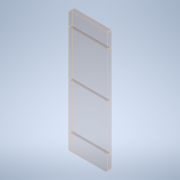
# Autodesk Inventor part: 関節3_上板
Saved by Autodesk Inventor 2021 (Build 250183000, 183)
## iProperties
Created: 2022-02-02
Part Number: 関節3_上板
Material: ポリカーボネート、スモーク
Document SubType Name: Modeling
Designer: hirohumi
Density: 1.2 g/cm^3
Appearance: ポリカーボネート - スモーク
Author: hirohumi
Autodesk Inventor part; units mm, degrees
ref_plane "YZ Plane" through (0, 0, 0) normal (1, 0, 0) x (0, 1, 0)
ref_plane "XZ Plane" through (0, 0, 0) normal (0, 1, 0) x (-1, 0, 0)
ref_plane "XY Plane" through (0, 0, 0) normal (0, 0, 1) x (1, 0, 0)
sketch "スケッチ1" plane through (0, 0, 0) normal (0, 0, 1) x (1, 0, 0)
  line L0 (25.5, 80) -> (-25.5, 80)
  line L1 (-25.5, 80) -> (-25.5, 60.7746)
  line L2 (-25.5, -80) -> (25.5, -80)
  line L3 (25.5, -80) -> (25.5, -60.7746)
  line L4 (25.5, 80) -> (-25.5, -80) construction
  line L5 (-25.5, 80) -> (25.5, -80) construction
  arc A0 (-25.5, 0.7746) -> (-25.5, -0.7746) centre (-26.9, 0) ccw construction
  arc A1 (-25.5, 60.7746) -> (-25.5, 59.2254) centre (-26.9, 60) ccw construction
  arc A2 (-25.5, -59.2254) -> (-25.5, -60.7746) centre (-26.9, -60) ccw construction
  arc A3 (25.5, 0.7746) -> (25.5, -0.7746) centre (26.9, 0) ccw
  arc A4 (25.5, 60.7746) -> (25.5, 59.2254) centre (26.9, 60) ccw
  arc A5 (25.5, -60.7746) -> (25.5, -59.2254) centre (26.9, -60) ccw construction
  arc A6 (-25.5, 59.2254) -> (-25.5, 60.7746) centre (-26.9, 60) ccw
  line L6 (-25.5, 60.7746) -> (-25.5, 59.2254) construction
  line L7 (-25.5, 59.2254) -> (-25.5, 0.7746)
  arc A7 (-25.5, -0.7746) -> (-25.5, 0.7746) centre (-26.9, 0) ccw
  line L8 (-25.5, -0.7746) -> (-25.5, -59.2254)
  line L9 (-25.5, 0.7746) -> (-25.5, -0.7746) construction
  line L10 (-25.5, -59.2254) -> (-25.5, -60.7746) construction
  line L11 (-25.5, -60.7746) -> (-25.5, -80)
  arc A8 (-25.5, -60.7746) -> (-25.5, -59.2254) centre (-26.9, -60) ccw
  arc A9 (25.5, -59.2254) -> (25.5, -60.7746) centre (26.9, -60) ccw
  line L12 (25.5, -60.7746) -> (25.5, -59.2254) construction
  line L13 (25.5, -59.2254) -> (25.5, -0.7746)
  arc A10 (25.5, -0.7746) -> (25.5, 0.7746) centre (26.9, 0) ccw construction
  line L14 (25.5, -0.7746) -> (25.5, 0.7746) construction
  line L15 (25.5, 0.7746) -> (25.5, 59.2254)
  arc A11 (25.5, 59.2254) -> (25.5, 60.7746) centre (26.9, 60) ccw construction
  line L16 (25.5, 59.2254) -> (25.5, 60.7746) construction
  line L17 (25.5, 60.7746) -> (25.5, 80)
  point P0 (0, 0)
  point P1 (0, 0)
  point P2 (0, 0)
  dimension "d0" = 51
  dimension "d1" = 160
  dimension "d2" = 3.2
  dimension "d3" = 3.2
  dimension "d4" = 3.2
  dimension "d5" = 60
  dimension "d6" = 60
  dimension "d7" = 3.2
  dimension "d8" = 3.2
  dimension "d9" = 3.2
  dimension "d10" = 60
  dimension "d11" = 60
  dimension "d12" = 1.4
  dimension "d13" = 1.4
  constraints: 50 parallel, 36 end point, 24 point on circle, 12 centre point, 7 perpendicular, 4 midpoint, 4 point on line, 4 vertical alignment, 2 horizontal alignment, 1 horizontal
  measures "d0" distance of L2.end L2.start
  measures "d1" distance of L2.start L0.end
  measures "d2" diameter of A0
  measures "d3" diameter of A1
  measures "d4" diameter of A2
  measures "d5" distance of A0.centre A1.centre
  measures "d6" distance of A2.centre A0.centre
  measures "d7" diameter of A3
  measures "d8" diameter of A4
  measures "d9" diameter of A5
  measures "d10" distance of A3.centre A4.centre
  measures "d11" distance of A5.centre A3.centre
  measures "d12" distance from line of L1 A0.centre
  measures "d13" distance from line of L3 A3.centre
extrude "押し出し1" add sketch "スケッチ1" along normal blind 6
sketch "スケッチ2" plane through (25.5, 0.7746, 0) normal (1, 0, 0) x (0, 0, -1)
  circle A0 centre (-3, -0.7746) radius 1.25
  circle A1 centre (-3, 59.2254) radius 1.25
  circle A2 centre (-3, -60.7746) radius 1.25
  point P0 (0, -0.7746)
  dimension "d16" = 2.5
  dimension "d17" = 2.5
  dimension "d18" = 2.5
  dimension "d19" = 60
  dimension "d20" = 60
  dimension "d21" = 3
  constraints: 3 centre point, 2 vertical alignment, 1 horizontal alignment
  measures "d16" diameter of A0
  measures "d17" diameter of A1
  measures "d18" diameter of A2
  measures "d19" distance of A0.centre A1.centre
  measures "d20" distance of A2.centre A0.centre
  measures "d21" distance of A0.centre point (0, -0.775)
extrude "押し出し2" cut sketch "スケッチ2" against normal through all
fillet "フィレット1" radius 2 4 edges at (25.5, 80, 3) (-25.5, 80, 3) (25.5, -80, 3) (-25.5, -80, 3)
